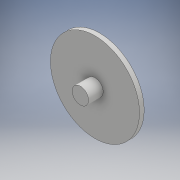
# Autodesk Inventor part: Motor_and_rotor
Saved by Autodesk Inventor 2018 (Build 220112000, 112)
## iProperties
Created: 2017-12-31
Part Number: Motor_and_rotor
Material: Generic
Document SubType Name: Modeling
Designer: suchanek
Density: 1 g/cm^3
Appearance: Default
Author: suchanek
Autodesk Inventor part; units mm, degrees
ref_plane "YZ Plane" through (0, 0, 0) normal (1, 0, 0) x (0, 1, 0)
ref_plane "XZ Plane" through (0, 0, 0) normal (0, 1, 0) x (-1, 0, 0)
ref_plane "XY Plane" through (0, 0, 0) normal (0, 0, 1) x (1, 0, 0)
sketch "Sketch1" plane through (0, 0, 0) normal (0, 0, 1) x (1, 0, 0)
  line L0 (0, 0) -> (7, 0)
  line L1 (7, 0) -> (7, 12.5)
  line L2 (7, 12.5) -> (0, 12.5)
  line L3 (0, 12.5) -> (0, 0)
  line L4 (0, 12.5) -> (38, 12.5)
  line L5 (38, 12.5) -> (38, 16.5)
  line L6 (38, 16.5) -> (0, 16.5)
  line L7 (0, 16.5) -> (0, 12.5)
  dimension "d0" = 7
  dimension "d1" = 12.5
  dimension "d2" = 38
  dimension "d3" = 4
  constraints: 16 end point, 4 parallel, 2 horizontal, 2 perpendicular
  measures "d0" distance of L2.end L1.end
  measures "d1" distance of L1.end L0.end
  measures "d2" distance of L6.end L5.end
  measures "d3" distance of L5.end L4.end
revolve "Revolution1" add sketch "Sketch1" angle 360 about axis through (0, 16.5, 0) along (0, -1, 0)
body "Solid1"
